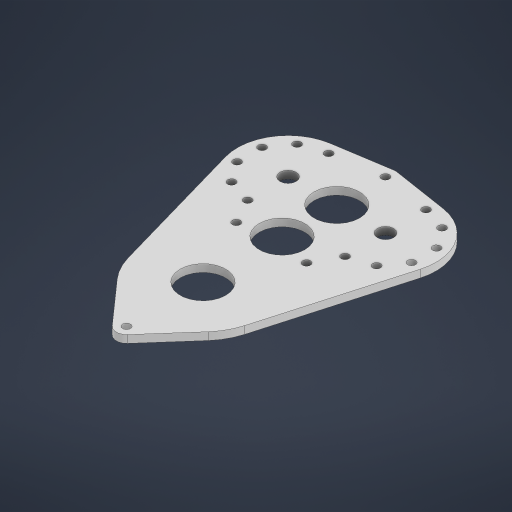
# Autodesk Inventor part: Gearbox4_001_Plate
Saved by Autodesk Inventor 2024.4 (Build 284460000, 460)
## iProperties
Created: 2026-06-11
Part Number: Gearbox4_001_Plate
Material: Generic
Document SubType Name: Modeling
Designer: stanr
Density: 1 g/cm^3
Appearance: Default
Author: stanr
Autodesk Inventor part; units mm, degrees
ref_plane "YZ Plane" through (0, 0, 0) normal (1, 0, 0) x (0, 1, 0)
ref_plane "XZ Plane" through (0, 0, 0) normal (0, 1, 0) x (-1, 0, 0)
ref_plane "XY Plane" through (0, 0, 0) normal (0, 0, 1) x (1, 0, 0)
sketch "Sketch3" plane through (0, 0, 0) normal (0, 1, 0) x (-1, 0, 0)
  circle A0 centre (0, 0) radius 22.86 construction
  circle A1 centre (30.5562, 0) radius 5.08
  circle A2 centre (-30.5562, 0) radius 5.08
  circle A3 centre (30.5562, 0) radius 8.89 construction
  circle A4 centre (-30.5562, 0) radius 8.89 construction
  circle A5 centre (0, 0) radius 14.2875
  circle A6 centre (-30.5562, 0) radius 31.75
  circle A7 centre (30.5562, 0) radius 31.75
  circle A8 centre (30.5562, -25.4) radius 2.4892
  circle A9 centre (45.4859, -20.549) radius 2.4892
  circle A10 centre (54.713, -7.849) radius 2.4892
  circle A11 centre (54.713, 7.849) radius 2.4892
  circle A12 centre (45.4859, 20.549) radius 2.4892
  circle A13 centre (30.5562, 25.4) radius 2.4892
  circle A14 centre (-30.5562, -25.4) radius 2.4892
  circle A15 centre (-45.4859, -20.549) radius 2.4892
  circle A16 centre (-54.713, -7.849) radius 2.4892
  circle A17 centre (-54.713, 7.849) radius 2.4892
  circle A18 centre (-45.4859, 20.549) radius 2.4892
  circle A19 centre (-30.5562, 25.4) radius 2.4892
  circle A20 centre (0, 34.3662) radius 11.43 construction
  circle A21 centre (0, 34.3662) radius 14.2875
  circle A22 centre (0, 83.9724) radius 38.1
  circle A23 centre (0, 83.9724) radius 14.2875
  circle A24 centre (22.0285, 41.0332) radius 6.35 construction
  circle A25 centre (22.0285, 41.0332) radius 2.4892
  line L0 (23.3206, 34.8161) -> (24.0958, 31.0858) construction
  line L1 (19.13, 46.6831) -> (17.3909, 50.0731) construction
  circle A26 centre (-22.0285, 41.0332) radius 6.35 construction
  circle A27 centre (-22.0285, 41.0332) radius 2.4892
  line L2 (-23.3206, 34.8161) -> (-24.0958, 31.0858) construction
  line L3 (-19.13, 46.6831) -> (-17.3909, 50.0731) construction
  circle A28 centre (0, 131.9012) radius 6.35
  circle A29 centre (0, 131.9012) radius 2.4892
  line L4 (1.4331, 125.715) -> (2.2929, 122.0033) construction
  line L5 (-1.4331, 125.715) -> (-2.2929, 122.0033) construction
  circle A30 centre (0, -30.5095) radius 2.4892
  circle A31 centre (0, -30.5095) radius 6.35
  line L6 (4.4867, -26.016) -> (8.0761, -22.4211) construction
  line L7 (-8.0884, -22.4335) -> (-4.4935, -26.0228) construction
  line L8 (4.7569, 136.1077) -> (28.5413, 109.2114)
  line L9 (-4.7569, 136.1077) -> (-28.5413, 109.2114)
  line L10 (-36.6386, 94.4235) -> (-61.0883, 8.7092)
  line L11 (35.4816, -31.3656) -> (0.9851, -36.7826)
  line L12 (-0.9851, -36.7826) -> (-35.4816, -31.3656)
  line L13 (61.0883, 8.7092) -> (36.6386, 94.4235)
  dimension "d159" = 76.2
  dimension "d137" = 45.72
  dimension "d138" = 10.16
  dimension "d140" = 17.78
  dimension "d141" = 28.575
  dimension "d142" = 30.5562
  dimension "d143" = 30.5562
  dimension "d144" = 63.5
  dimension "d145" = 63.5
  dimension "d146" = 4.9784
  dimension "d147" = 25.4
  dimension "d150" = 180
  dimension "d154" = 180
  dimension "d156" = 22.86
  dimension "d158" = 34.3662
  dimension "d160" = 49.6062
  dimension "d161" = 28.575
  dimension "d162" = 12.7
  dimension "d163" = 4.9784
  dimension "d166" = 3.81
  dimension "d167" = 5.08
  constraints: 31 centre point, 28 end point, 20 point on circle, 15 point on line, 12 coincident, 10 equal radius, 8 tangent, 5 equal length, 5 vertical alignment, 3 horizontal alignment, 1 perpendicular, 36 other
  measures "d137" diameter of A0
  measures "d138" diameter of A1
  measures "d140" diameter of A3
  measures "d141" diameter of A5
  measures "d142" distance of A1.centre A5.centre
  measures "d143" distance of A5.centre A2.centre
  measures "d144" diameter of A6
  measures "d145" diameter of A7
  measures "d146" diameter of A8
  measures "d147" distance of A1.centre A8.centre
  measures "d156" diameter of A20
  measures "d158" distance of point (0, 0) A20.centre
  measures "d160" distance of A20.centre point (0, 83.972)
  measures "d161" diameter of A23
  measures "d162" diameter of A24
  measures "d163" diameter of A25
  measures "d166" distance of L3.start L3.end
  measures "d167" distance of L6.start L6.end
extrude "Extrusion2" add sketch "Sketch3" along normal blind 4.7625 contours A5 A7 A21 | A5 A6 A21 A7 | A7 L11 A31 L12 A6 A5 | A5 A6 A21 | A21 A22 L13 A7 | A31 | A6 L10 A22 A21 | A22 A21 | A22 L9 A28 L8 | A28 picked at (-8.1813, 55.8072)
body "Solid2"
